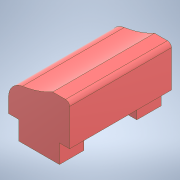
# Autodesk Inventor part: 103.020.01_Positionsausgleich
Saved by Autodesk Inventor 2021 (Build 250183000, 183)
## iProperties
Created: 2021-12-04
Part Number: 103.020.01_Positionsausgleich
Material: Polypropylen
Document SubType Name: Modeling
Designer: Sebastian Seewald
Density: 0.899 g/cm^3
Appearance: Glatt - Esche
Mass: 4.02907 g
Surface Area: 19.8395 cm^2
Volume: 4.48172 cm^3
Author: Sebastian Seewald
Autodesk Inventor part; units mm, degrees
ref_plane "YZ Plane" through (0, 0, 0) normal (1, 0, 0) x (0, 1, 0)
ref_plane "XZ Plane" through (0, 0, 0) normal (0, 1, 0) x (-1, 0, 0)
ref_plane "XY Plane" through (0, 0, 0) normal (0, 0, 1) x (1, 0, 0)
sketch "Skizze1" plane through (0, 0, 0) normal (0, 0, 1) x (1, 0, 0)
  circle A0 centre (0, 0) radius 22.75
  line L0 (0, -22.75) -> (0, -30)
  line L1 (0, -30) -> (15, -30)
  line L2 (15, -30) -> (15, -17.1045)
  line L3 (7.5, -17.7699) -> (7.5, -35.7566) construction
  line L4 (10.8426, -20) -> (15, -20)
  point P0 (7.5, -21.4782)
  dimension "d0" = 45.5
  dimension "d1" = 15
  dimension "d2" = 0
  dimension "d3" = 7.5
  dimension "d27" = 30
  dimension "d28" = 10
  constraints: 10 end point, 4 point on circle, 3 perpendicular, 2 point on line, 2 vertical, 1 centre point, 1 coincident
  measures "d0" diameter of A0
  measures "d1" distance between parallel lines of L0 L2
  measures "d2" distance from line of L0 point (0, 0)
  measures "d3" distance between parallel lines of L0 L3
  measures "d27" distance from line of L1 point (0, 0)
  measures "d28" distance between parallel lines of L1 L4
extrude "Extrusion1" add sketch "Skizze1" along normal blind 25 contours A0 L4 L2 L1 L0
fillet "Rundung1" radius 4 1 edges at (0, -22.75, 12.5)
sketch "Skizze2" plane through (0, -30, 0) normal (0, -1, 0) x (1, 0, 0)
  line L0 (2.5, 25) -> (12.5, 25)
  line L1 (12.5, 25) -> (12.5, 19)
  line L2 (12.5, 19) -> (2.5, 19)
  line L3 (2.5, 19) -> (2.5, 25)
  line L4 (2.5, 6) -> (12.5, 6)
  line L5 (12.5, 6) -> (12.5, 0)
  line L6 (12.5, 0) -> (2.5, 0)
  line L7 (2.5, 0) -> (2.5, 6)
  line L8 (7.5, 27.4511) -> (7.5, -5.4268) construction
  line L9 (0, 0) -> (0, 25) projected
  line L10 (0, 25) -> (15, 25) projected
  line L11 (0, 0) -> (15, 0) projected
  dimension "d8" = 6
  dimension "d9" = 6
  dimension "d10" = 10
  dimension "d11" = 7.5
  constraints: 18 end point, 4 parallel, 2 collinear, 2 horizontal, 2 perpendicular, 2 point on line, 1 vertical, 1 other
  measures "d8" distance of L2.end L0.start
  measures "d9" distance of L6.end L4.start
  measures "d10" distance of L0.start L0.end
  measures "d11" distance between parallel lines of L9 L8
extrude "Extrusion2" add sketch "Skizze2" along normal blind 5
sketch "Skizze3" plane through (0, -30, 0) normal (0, -1, 0) x (1, 0, 0)
  line L0 (0, 0) -> (0, 25) projected
  line L1 (2.5, 0) -> (12.5, 0) projected
  point P0 (7.5, 12.5)
  dimension "d25" = 7.5
  dimension "d26" = 12.5
  measures "d25" distance from line of L0 point (7.5, 12.5)
  measures "d26" distance from line of L1 point (7.5, 12.5)
hole "Bohrung1" at (7.5, -30, 12.5) direction (0, 1, 0) diameter 2.459 depth 6 tip angle 118 thread size "M3x0.5" class "6H" standard "ISO Metric profile"
fillet "Rundung2" radius 1 1 edges at (15, -20, 12.5)
chamfer "Fase1" distance 0.4 angle 45 8 edges at (7.5, -35, 25) (2.5, -35, 22) (7.5, -35, 19) (12.5, -35, 22) (12.5, -35, 3) (7.5, -35, 6) (2.5, -35, 3) (7.5, -35, 0)
